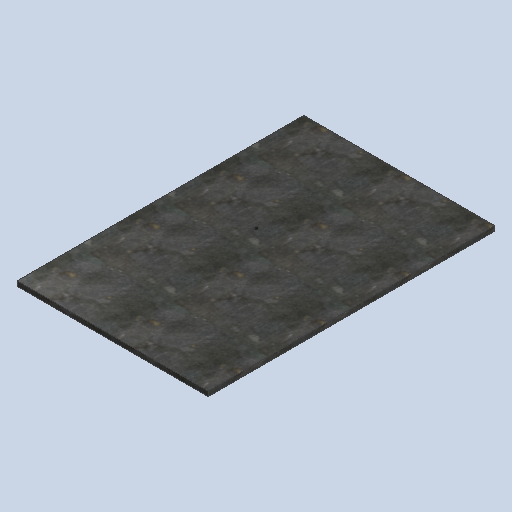
# Autodesk Inventor part: PlaqueSupport
Saved by Autodesk Inventor 2025.4 (Build 294407000, 407)
## iProperties
Created: 2020-04-21
Part Number: PlaqueSupport
Material: Steel
Document SubType Name: Modeling
Designer: Mathieu
Density: 7.85 g/cm^3
Appearance: Plate
Author: Mathieu
Autodesk Inventor part; units mm, degrees
ref_plane "YZ Plane" through (0, 0, 0) normal (1, 0, 0) x (0, 1, 0)
ref_plane "XZ Plane" through (0, 0, 0) normal (0, 1, 0) x (-1, 0, 0)
ref_plane "XY Plane" through (0, 0, 0) normal (0, 0, 1) x (1, 0, 0)
sketch "Sketch1" plane through (0, 0, 0) normal (0, 1, 0) x (-1, 0, 0)
  line L0 (-200, -300) -> (200, -300)
  line L1 (200, -300) -> (200, 300)
  line L2 (200, 300) -> (-200, 300)
  line L3 (-200, 300) -> (-200, -300)
  line L4 (-200, -300) -> (200, 300) construction
  line L5 (200, -300) -> (-200, 300) construction
  point P0 (0, 0)
  dimension "d0" = 600
  dimension "d1" = 400
  constraints: 12 end point, 2 midpoint, 2 parallel, 1 horizontal, 1 perpendicular
  measures "d0" distance of L0.end L1.end
  measures "d1" distance of L1.end L2.end
extrude "Extrusion1" add sketch "Sketch1" along normal blind 10
sketch "Sketch2" plane through (0, 0, 0) normal (0, -1, 0) x (1, 0, 0)
  point P0 (-45, -45)
hole "Hole1" at (-45, 0, -45) direction (0, 1, 0) diameter 9 end through all
body "Solid1"
